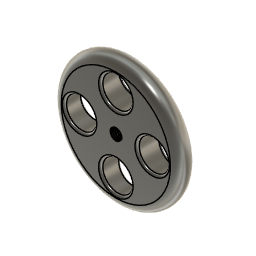
rotator wheel v5 (Autodesk Fusion 360 design; units mm, degrees)
Autodesk Fusion 360 part; units mm, degrees
sketch "outline" plane through (0, 0, 0) normal (0, 0, 1) x (1, 0, 0)
  line L0 (0, 0) -> (36, 0)
  arc A0 (36, 0) -> (36, 12) centre (36, 6) ccw
  line L1 (36, 12) -> (8, 16)
  line L2 (8, 16) -> (0, 16)
  line L3 (0, 16) -> (0, 0)
  dimension "d1" = 36
  dimension "d2" = 12
  dimension "d3" = 16
  dimension "d4" = 8
  dimension "d5" = 6
  constraint coincident L0.start L3.end
  constraint horizontal L0
  constraint tangent L0 A0
  constraint horizontal L2
  constraint perpendicular L0 L3
  measures "d1" distance of L0.start L0.end
  measures "d2" distance of L0.end A0.end
  measures "d3" distance of L0.start L2.end
  measures "d4" distance of L1.end L2.end
  measures "d5" radius of A0
revolve "Revolve1" add sketch "outline" angle 360 about axis through (0, 16, 0) along (0, -1, 0)
hole "Hole1" at (0, 16, 0) direction (0, -1, 0) diameter 6.78 end through all
thread "Thread1" "ISO Metric profile 8.0 M8x1.25 6H" major diameter 8.17 minor diameter 6.7795 pitch 1.25 angle 60 modelled right hand crest width 0.343 on face at (0.3375, 10.6667, 3.3732) crest through (0, 15.6875, 3.3898)
sketch "finger hole" plane through (0, 0, 0) normal (0, -1, 0) x (1, 0, 0)
  spline S0 degree 3 poles (-0.2131, 4.0794) (0.3083, 4.0628) (0.8216, 3.946) (1.7575, 3.5264) (2.1736, 3.2337) (2.8561, 2.5153) (3.1205, 2.1013) (3.4665, 1.21) (3.5508, 0.7439) (3.5364, -0.0031) (3.4983, -0.2795) (3.3583, -0.8109) (3.2584, -1.0645) (3.1292, -1.3034) knots 0 0 0 0 0.15651 0.15651 0.307908 0.307908 0.454192 0.454192 0.595358 0.595358 0.679011 0.679011 0.76076 0.76076 0.76076 0.76076
  arc A0 (-1.7654, -2.8937) -> (3.1292, -1.3034) centre (0, 0) ccw
  spline S1 degree 3 poles (-1.7654, -2.8937) (-2.1691, -2.7005) (-2.5303, -2.4289) (-3.1424, -1.7518) (-3.3826, -1.3484) (-3.7037, -0.4568) (-3.7754, 0.0249) (-3.7327, 1.0064) (-3.612, 1.4963) (-3.2703, 2.236) (-3.1042, 2.5046) (-2.7085, 3.0023) (-2.4791, 3.2286) (-2.2254, 3.4256) knots 0 0 0 0 0.134259 0.134259 0.273621 0.273621 0.418082 0.418082 0.567642 0.567642 0.661748 0.661748 0.757764 0.757764 0.757764 0.757764
  arc A1 (-0.2131, 4.0794) -> (-2.2254, 3.4256) centre (0, 0) ccw
  circle A2 centre (0, 0) radius 36
  circle A3 centre (0, -24) radius 10
  dimension "d12" = 20
  dimension "d13" = 24
  measures "d12" diameter of A3
  measures "d13" distance of A0.centre A3.centre
extrude "Extrude1" cut sketch "finger hole" against normal through all contours A3
fillet "Fillet1" radius 1.4 2 edges at (-8.9741, 12.8869, -28.4074) (-9.3233, 0, -20.3838)
pattern_circular "C-Pattern1" count 4 over 360 about axis through (0, 1.75, 0) along (0, 1, 0) of "Extrude1", "Fillet1"
named bodies: "rotator wheel"
